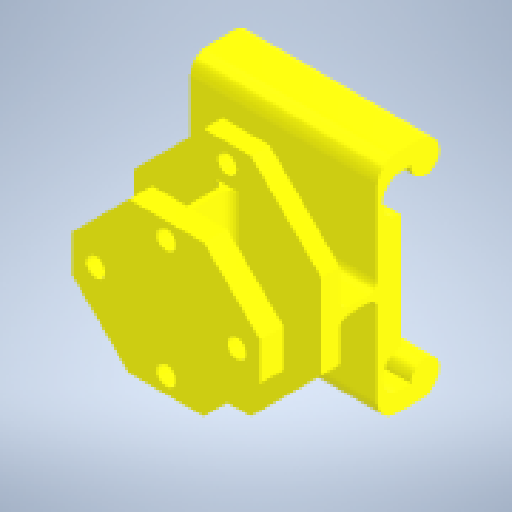
# Autodesk Inventor part: MicroRail-FlextureBase
Saved by Autodesk Inventor 2023.1 (Build 271208000, 208)
## iProperties
Created: 2023-06-05
Part Number: MicroRail-FlextureBase
Material: ABS Plastic
Document SubType Name: Modeling
Designer: hello
Density: 1.06 g/cm^3
Appearance: Smooth - Yellow
Mass: 24.8987 g
Surface Area: 148.331 cm^2
Volume: 23.4894 cm^3
Author: hello
Autodesk Inventor part; units mm, degrees
ref_plane "YZ Plane" through (0, 0, 0) normal (1, 0, 0) x (0, 1, 0)
ref_plane "XZ Plane" through (0, 0, 0) normal (0, 1, 0) x (-1, 0, 0)
ref_plane "XY Plane" through (0, 0, 0) normal (0, 0, 1) x (1, 0, 0)
sketch "Sketch1" plane through (0, 0, 0) normal (1, 0, 0) x (0, 1, 0)
  line L0 (-24, -4.205) -> (-24, 1)
  line L1 (-20, 5) -> (20, 5)
  line L2 (24, 1) -> (24, -4.205)
  line L3 (20, -8.205) -> (19.9, -8.205)
  line L4 (-20, -8.205) -> (-19.9, -8.205)
  line L5 (-20.15, -2.2154) -> (-20.15, 0)
  line L6 (-20.15, 0) -> (20.15, 0)
  line L7 (20.15, 0) -> (20.15, -2.2154)
  line L8 (-0.625, 5) -> (-0.625, 13)
  line L9 (-0.625, 13) -> (0.625, 13)
  line L10 (0.625, 13) -> (0.625, 5)
  line L11 (-24, 17) -> (24, 17)
  line L12 (24, 17) -> (24, 13)
  line L13 (24, 13) -> (-24, 13)
  line L14 (-24, 13) -> (-24, 17)
  arc A0 (24, 1) -> (20, 5) centre (20, 1) ccw
  arc A1 (-20, 5) -> (-24, 1) centre (-20, 1) ccw
  arc A2 (20.15, 0) -> (13.15, 0) centre (16.65, 0) ccw
  arc A3 (-13.15, 0) -> (-20.15, 0) centre (-16.65, 0) ccw
  arc A4 (20.15, -2.2154) -> (19.9, -8.205) centre (19.9, -5.205) ccw
  arc A5 (20, -8.205) -> (24, -4.205) centre (20, -4.205) ccw
  circle A6 centre (-19.9, -5.205) radius 3
  arc A7 (-24, -4.205) -> (-20, -8.205) centre (-20, -4.205) ccw
  point P0 (0, 0)
  point P1 (-24, -8.205)
  point P2 (-24, 5)
  point P3 (24, 5)
  point P4 (24, -8.205)
  point P5 (0, 5)
  point P6 (0, 0)
  point P7 (0, 13)
  point P8 (0.625, 13)
  point P9 (-0.625, 13)
  dimension "d65" = 6
  dimension "d2" = 40.3
  dimension "d10" = 48
  dimension "d11" = 5
  dimension "d13" = 1.25
  dimension "d14" = 8
  dimension "d15" = 4
  dimension "d52" = 4
  dimension "d53" = 7
  dimension "d54" = 7
  dimension "d61" = 6
  dimension "d62" = 5.205
  dimension "d63" = 0.25
  dimension "d64" = 4
  dimension "d66" = 0.25
  dimension "d67" = 4
  constraints: 30 end point, 15 point on line, 14 point on circle, 8 perpendicular, 8 tangent, 7 centre point, 5 vertical alignment, 4 midpoint, 3 parallel, 2 horizontal, 2 vertical, 1 coincident, 1 equal radius, 1 horizontal alignment, 3 other
  measures "d2" distance of L5.end L6.end
  measures "d10" distance of point (-24, 5) point (24, 5)
  measures "d11" distance between parallel lines of L1 L6
  measures "d13" distance of L8.end L9.end
  measures "d14" distance of L8.start L8.end
  measures "d15" distance of L13.end L11.start
  measures "d52" radius of A0
  measures "d53" distance of A2.end L6.end
  measures "d54" distance of L5.end A3.start
  measures "d61" diameter of A4
  measures "d62" distance from line of L6 A4.centre
  measures "d63" distance from line of L7 A4.centre
  measures "d64" radius of A5
  measures "d66" distance from line of L5 point (-19.9, -5.205)
  measures "d67" radius of A7
extrude "Extrusion1" add sketch "Sketch1" along normal mid plane 40 contours L0 A1 L1 A0 L2 A5 L3 A4 L7 A2 L6 A3 L5 A6 A7 | A6 L4 | L8 L9 L10 L1 | L13 L14 L11 L12 L9
sketch "Sketch2" plane through (-20, -24, 17) normal (0, 0, 1) x (1, 0, 0)
  line L0 (0, 0) -> (40, 0) projected
  line L1 (40, 48) -> (40, 0) projected
  line L2 (0, 48) -> (40, 48) projected
  line L3 (0, 0) -> (0, 48) projected
  line L4 (20.625, 8) -> (19.375, 8)
  line L5 (19.375, 8) -> (19.375, 40)
  line L6 (19.375, 40) -> (20.625, 40)
  line L7 (20.625, 40) -> (20.625, 8)
  line L8 (20.625, 8) -> (19.375, 40) construction
  line L9 (19.375, 8) -> (20.625, 40) construction
  point P0 (20, 24)
  point P1 (20.75, 0)
  point P2 (20.75, 50)
  point P3 (19.25, 50)
  point P4 (19.25, 0)
  point P5 (20, 8)
  dimension "d16" = 1.25
  dimension "d19" = 8
  constraints: 12 end point, 3 midpoint, 2 parallel, 1 horizontal, 1 perpendicular
  measures "d16" distance of L4.start L4.end
  measures "d19" distance from line of L0 point (20, 8)
extrude "Extrusion2" add sketch "Sketch2" along normal blind 8 contours L4 L5 L6 L7
sketch "Sketch3" plane through (-20, -24, 17) normal (0, 0, 1) x (1, 0, 0)
  line L0 (20.625, 40) -> (20.625, 8) projected
  line L1 (20.625, 8) -> (19.375, 8) projected
  line L2 (19.375, 8) -> (19.375, 40) projected
  line L3 (19.375, 40) -> (20.625, 40) projected
  line L4 (0, 0) -> (40, 0) projected
  line L5 (40, 48) -> (40, 0) projected
  line L6 (0, 48) -> (40, 48) projected
  line L7 (0, 0) -> (0, 48) projected
  line L8 (20.625, 8) -> (19.375, 8) projected
  line L9 (20, 8) -> (20, 0)
  line L10 (19.375, 40) -> (20.625, 40) projected
  line L11 (20, 40) -> (20, 48)
  point P0 (20, 24)
  point P1 (20, 4)
  point P2 (20, 44)
  constraints: 6 midpoint, 4 end point
hole "Hole1" at (0, -20, 17) at (0, 20, 17) direction (0, 0, -1) diameter 4 depth 8 tip angle 118
sketch "Sketch4" plane through (-20, -24, 25) normal (0, 0, 1) x (1, 0, 0)
  line L0 (0, 8) -> (40, 8)
  line L1 (40, 8) -> (40, 40)
  line L2 (40, 40) -> (0, 40)
  line L3 (0, 40) -> (0, 8)
  line L4 (0, 8) -> (40, 40) construction
  line L5 (40, 8) -> (0, 40) construction
  line L6 (20.625, 40) -> (19.375, 40) projected
  line L7 (0, 0) -> (0, 48) projected
  point P0 (20, 24)
  point P1 (20, 40)
  point P2 (0, 24)
  constraints: 12 end point, 6 midpoint, 2 parallel, 1 horizontal, 1 perpendicular
extrude "Extrusion3" add sketch "Sketch4" along normal blind 5
sketch "Sketch5" plane through (-20, -24, 30) normal (0, 0, 1) x (1, 0, 0)
  line L0 (40, 40) -> (0, 40) projected
  line L1 (0, 40) -> (0, 8) projected
  line L2 (0, 8) -> (40, 8) projected
  line L3 (40, 8) -> (40, 40) projected
  line L4 (5, 24) -> (35, 24)
  point P0 (20, 24)
  point P1 (20, 24)
  dimension "d29" = 5
  constraints: 3 coincident, 2 end point, 1 horizontal, 1 midpoint
  measures "d29" distance from line of L1 L4.start
hole "Hole2" at (-15, 0, 30) at (15, 0, 30) direction (0, 0, -1) diameter 4 depth 8 tip angle 118
sketch "Sketch6" plane through (-20, -24, 30) normal (0, 0, 1) x (1, 0, 0)
  circle A0 centre (5, 24) radius 2 projected
  circle A1 centre (35, 24) radius 2 projected
  line L0 (40, 40) -> (0, 40) projected
  line L1 (0, 40) -> (0, 8) projected
  line L2 (0, 8) -> (40, 8) projected
  line L3 (40, 8) -> (40, 40) projected
  line L4 (20, 11.5) -> (20, 36.5)
  point P0 (20, 24)
  point P1 (20, 24)
  point P2 (20, 24)
  dimension "d38" = 25
  constraints: 4 coincident, 2 end point, 1 midpoint, 1 vertical
  measures "d38" distance of L4.start L4.end
hole "Hole3" at (0, -12.5, 30) at (0, 12.5, 30) direction (0, 0, -1) diameter 4 depth 5
chamfer "Chamfer1" distance 15 angle 45 4 edges at (-20, -24, 15) (-20, 24, 15) (20, -24, 15) (20, 24, 15)
chamfer "Chamfer2" distance 12 angle 45 4 edges at (20, 16, 27.5) (20, -16, 27.5) (-20, -16, 27.5) (-20, 16, 27.5)
fillet "Fillet1" radius 2 6 edges at (0.625, 0, 17) (-0.625, 0, 17) (0, -0.625, 5) (0, 0.625, 5) (0, -0.625, 13) (0, 0.625, 13)
equation "\"d54\" = d53"
equation "\"d66\" = d63"
body "Solid1"
